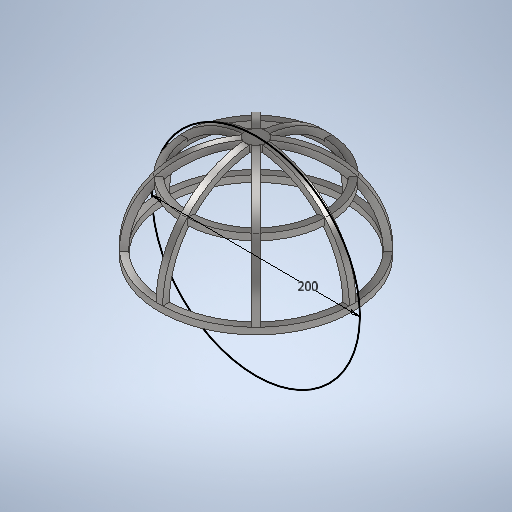
# Autodesk Inventor part: Dome
Saved by Autodesk Inventor 2025.1 (Build 291241000, 241)
## iProperties
Created: 2024-11-09
Part Number: Dome
Material: Steel, Mild
Document SubType Name: Modeling
Designer: monos
Density: 7.85 g/cm^3
Appearance: Semi-Polished
Mass: 646.174 g
Surface Area: 503.809 cm^2
Volume: 82.3152 cm^3
Author: monos
Autodesk Inventor part; units mm, degrees
sketch "200mm Measuring Ring" plane through (0, 0, 0) normal (0, 0, 1) x (1, 0, 0)
  circle A0 centre (0, 0) radius 100
  dimension "d4" = 200
  constraints: 1 centre point, 1 coincident
  measures "d4" diameter of A0
sketch "Sketch1" plane through (0, 0, 0) normal (0, 1, 0) x (-1, 0, 0)
  circle A0 centre (0, 0) radius 93
  circle A1 centre (0, 0) radius 86.65
  dimension "d0" = 186
  dimension "d1" = 173.3
  constraints: 2 centre point, 2 coincident
  measures "d0" diameter of A0
  measures "d1" diameter of A1
extrude "Extrusion1" add sketch "Sketch1" along normal blind 6.35
sketch "Sketch3" plane through (0, 0, 0) normal (1, 0, 0) x (0, 1, 0)
  line L0 (6.35, -93) -> (6.35, 93) projected
  arc A0 (99.35, 0) -> (6.35, 93) centre (6.35, 0) ccw
  line L1 (6.35, 0) -> (99.35, 0) construction
  line L2 (6.35, 0) -> (6.35, 93) construction
  arc A1 (93, 0) -> (6.35, 86.65) centre (6.35, 0) ccw
  arc A2 (6.35, -93) -> (99.35, 0) centre (6.35, 0) ccw
  arc A3 (6.35, -86.65) -> (93, 0) centre (6.35, 0) ccw
  line L3 (99.35, 0) -> (93, 0)
  line L4 (6.35, 93) -> (6.35, 86.65)
  line L5 (6.35, -93) -> (6.35, -86.65)
  line L6 (99.35, 0) -> (93, 0)
  point P0 (0, 0)
  point P1 (6.35, 86.65)
  dimension "d5" = 90
  dimension "d6" = 86.65
  dimension "d7" = 86.65
  constraints: 12 end point, 8 point on circle, 4 centre point, 4 collinear, 3 coincident, 3 point on line, 1 midpoint
  measures "d5" angle of L1 L2
  measures "d6" radius of A1
  measures "d7" radius of A3
extrude "Extrusion2" add sketch "Sketch3" along normal mid plane 6.35 contours L0 A3 L3 A2 | L3 A1 L0 A0
sketch "Sketch4" plane through (0, 0, 0) normal (0, 0, 1) x (1, 0, 0)
  line L0 (93, 6.35) -> (-93, 6.35) projected
  arc A0 (0, 99.35) -> (-93, 6.35) centre (0, 6.35) ccw
  arc A1 (0, 93) -> (-86.65, 6.35) centre (0, 6.35) ccw
  line L1 (-93, 6.35) -> (-86.65, 6.35)
  line L2 (0, 99.35) -> (0, 93)
  arc A2 (93, 6.35) -> (0, 99.35) centre (0, 6.35) ccw
  arc A3 (86.65, 6.35) -> (0, 93) centre (0, 6.35) ccw
  line L3 (0, 99.35) -> (0, 93)
  line L4 (86.65, 6.35) -> (93, 6.35)
  line L5 (93, 6.35) -> (86.65, 6.35)
  line L6 (-86.65, 6.35) -> (-93, 6.35)
  line L7 (0, 99.35) -> (0, 93)
  point P0 (0, 0)
  dimension "d8" = 86.65
  dimension "d9" = 86.65
  constraints: 14 end point, 8 point on circle, 4 centre point, 4 collinear, 3 coincident, 2 point on line, 1 horizontal, 1 midpoint, 1 perpendicular, 1 vertical
  measures "d8" radius of A1
  measures "d9" radius of A3
extrude "Extrusion3" add sketch "Sketch4" along normal mid plane 6.35 contours L0 A3 L2 A2 | L2 A1 L0 A0
ref_plane "Work Plane1" through (0, 0, 0) normal (-0.7071068, 0, 0.7071068) x (0, -1, 0)
sketch "Sketch5" plane through (0, 0, 0) normal (-0.7071068, 0, 0.7071068) x (0, -1, 0)
  line L0 (-6.35, -61.2311) -> (-6.35, 61.2311) projected
  line L1 (0, 93) -> (-6.35, 93) projected
  arc A0 (-6.35, 93) -> (-99.35, 0) centre (-6.35, 0) ccw
  line L2 (-6.35, 65.7212) -> (-6.35, -61.2708) projected
  arc A1 (-6.35, 86.65) -> (-93, 0) centre (-6.35, 0) ccw
  arc A2 (-99.35, 0) -> (-6.35, -93) centre (-6.35, 0) ccw
  arc A3 (-93, 0) -> (-6.35, -86.65) centre (-6.35, 0) ccw
  line L3 (-99.35, 0) -> (-93, 0)
  line L4 (-6.35, -93) -> (-6.35, -86.65)
  line L5 (-6.35, 86.65) -> (-6.35, 93)
  line L6 (0, 93) -> (0, -93) projected
  point P0 (0, 0)
  point P1 (-93, 0)
  point P2 (-6.35, 89.825)
  point P3 (-93, 0)
  dimension "d14" = 86.65
  dimension "d15" = 86.65
  constraints: 8 point on circle, 6 end point, 4 centre point, 3 coincident, 3 point on line, 1 horizontal, 1 midpoint, 1 parallel, 1 perpendicular
  measures "d14" radius of A1
  measures "d15" radius of A3
extrude "Extrusion4" add sketch "Sketch5" along normal mid plane 6.35
ref_plane "Work Plane3" through (0, 0, 0) normal (0.7071068, 0, 0.7071068) x (0, 1, 0)
sketch "Sketch7" plane through (0, 0, 0) normal (0.7071068, 0, 0.7071068) x (0, 1, 0)
  line L0 (6.35, 0) -> (6.35, -61.2708) projected
  line L1 (6.35, -93) -> (6.35, -67.9677) projected
  arc A0 (6.35, -93) -> (99.35, 0) centre (6.35, 0) ccw
  arc A1 (6.35, -86.65) -> (93, 0) centre (6.35, 0) ccw
  line L2 (6.35, 67.9677) -> (6.35, 93) projected
  arc A2 (99.35, 0) -> (6.35, 93) centre (6.35, 0) ccw
  arc A3 (93, 0) -> (6.35, 86.65) centre (6.35, 0) ccw
  line L3 (99.35, 0) -> (93, 0)
  line L4 (6.35, -93) -> (6.35, -86.65)
  line L5 (6.35, 93) -> (6.35, 86.65)
  point P0 (93, 0)
  point P1 (6.35, -86.65)
  point P2 (6.35, 86.65)
  dimension "d27" = 86.65
  dimension "d28" = 86.65
  constraints: 8 point on circle, 6 end point, 4 centre point, 3 coincident, 2 collinear, 1 horizontal
  measures "d27" radius of A1
  measures "d28" radius of A3
extrude "Extrusion7" add sketch "Sketch7" along normal mid plane 6.35
ref_plane "Top Disk" through (0, 99.35, 0) normal (0, 1, 0) x (1, 0, 0)
sketch "Sketch8" plane through (0, 99.35, 0) normal (0, 1, 0) x (1, 0, 0)
  line L0 (3.175, -1.3151) -> (0, 0) projected
  circle A0 centre (0, 0) radius 10
  dimension "d31" = 20
  constraints: 1 centre point, 1 coincident
  measures "d31" diameter of A0
extrude "Extrusion8" add sketch "Sketch8" against normal blind 6.35
ref_plane "Work Plane5" through (0, 65, 0) normal (0, 1, 0) x (-1, 0, 0)
sketch "Sketch9" plane through (0, 65, 0) normal (0, 1, 0) x (-1, 0, 0)
  line L0 (0, 0) -> (-7.6651, 3.175) projected
  circle A0 centre (0, 0) radius 69.5
  line L1 (3.175, -7.6651) -> (0, 0) projected
  circle A1 centre (0, 0) radius 63.15
  dimension "d35" = 139
  dimension "d36" = 126.3
  constraints: 2 centre point, 1 coincident
  measures "d35" diameter of A0
  measures "d36" diameter of A1
extrude "Middle ring" add sketch "Sketch9" along normal mid plane 6.35
body "Solid1"
